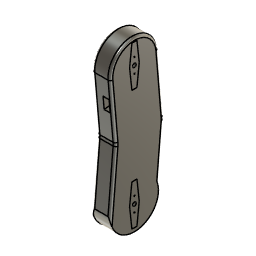
Lower-arm_segment (Autodesk Fusion 360 design; units mm, degrees)
Autodesk Fusion 360 part; units mm, degrees
note: some values were not read from the file. Chosen so that the rebuilt part matches the saved one: which face or edge a step refers to. Set by a fixed rule: which sketch regions a step uses.
sketch "Sketch1" plane through (0, 0, 0) normal (1, 0, 0) x (0, 1, 0)
  circle A0 centre (0, 0) radius 20
  circle A1 centre (0, 0) radius 1.5
  line L0 (0, 0) -> (4, 0)
  line L1 (0, 0) -> (-4, 0)
  line L2 (0, 0) -> (0, 17)
  line L3 (0, 17) -> (-2.1, 17)
  line L4 (0, 17) -> (2.1, 17)
  line L5 (-2.1, 17) -> (-4, 0)
  line L6 (2.1, 17) -> (4, 0)
  line L7 (-2.1, -17) -> (-4, 0)
  line L8 (0, -17) -> (2.1, -17)
  line L9 (0, -17) -> (-2.1, -17)
  line L10 (2.1, -17) -> (4, 0)
  line L11 (0, 0) -> (0, 6)
  line L12 (0, 0) -> (0, -6)
  circle A2 centre (0, 6) radius 0.5
  circle A3 centre (0, -6) radius 0.5
  line L13 (0, 0) -> (0, 8.5)
  line L14 (0, 0) -> (0, 100)
  line L15 (0, 0) -> (0, 50)
  line L16 (-6.3086, 50) -> (9.6914, 50)
  line L17 (2.1, 83) -> (4, 100)
  line L18 (0, 83) -> (2.1, 83)
  line L19 (0, 83) -> (-2.1, 83)
  line L20 (-2.1, 83) -> (-4, 100)
  line L21 (2.1, 117) -> (4, 100)
  line L22 (-2.1, 117) -> (-4, 100)
  line L23 (0, 117) -> (-2.1, 117)
  line L24 (0, 117) -> (2.1, 117)
  circle A4 centre (0, 100) radius 1.5
  circle A5 centre (0, 106) radius 0.5
  circle A6 centre (0, 94) radius 0.5
  circle A7 centre (0, 100) radius 20
  line L25 (-20, 0) -> (-15.741, 48.6808)
  line L26 (-20, 0) -> (10, 0) construction
  line L27 (20, 0) -> (24.261, 48.7037)
  line L28 (20, 0) -> (55, 0) construction
  line L29 (-19.9211, 98.2256) -> (-15.7431, 51.319)
  line L30 (19.9264, 101.7139) -> (24.2629, 51.2965)
  arc A8 (-15.741, 48.6808) -> (-15.7431, 51.319) centre (-30.6839, 49.9882) ccw
  arc A9 (24.261, 48.7037) -> (24.2629, 51.2965) centre (9.3181, 50.011) ccw
  line L31 (20, 0) -> (-20, 0)
  point P0 (-15.6256, 50)
  point P1 (24.3744, 50)
  dimension "d1" = 40
  dimension "d5" = 3
  dimension "d6" = 4
  dimension "d7" = 4
  dimension "d8" = 17
  dimension "d9" = 2.1
  dimension "d10" = 2.1
  dimension "d11" = 6
  dimension "d12" = 6
  dimension "d13" = 1
  dimension "d14" = 1
  dimension "d15" = 100
  dimension "d16" = 50
  dimension "d17" = 85
  dimension "d19" = 85
  dimension "d21" = 15
  dimension "d22" = 15
  constraint coincident A0.centre A1.centre
  constraint horizontal L0
  constraint parallel L0 L1
  constraint vertical L2
  constraint perpendicular L2 L3
  constraint perpendicular L2 L4
  constraint symmetric L6.end L0 L10.end
  constraint symmetric L0 L1.end L5.end
  constraint symmetric L0 L2.end L8.start
  constraint symmetric L0 L3.end L7.start
  constraint symmetric L0 L4.end L8.end
  constraint perpendicular L1 L11
  constraint perpendicular L1 L12
  constraint coincident L11.end A2.centre
  constraint coincident L12.end A3.centre
  constraint midpoint L2 L13.end
  constraint parallel L13 L14
  constraint parallel L14 L15
  constraint perpendicular L15 L16
  constraint coincident L15.end L16
  constraint symmetric A0 L16 A7
  constraint symmetric A1 L16 A4
  constraint symmetric L0.end L16 L17.end
  constraint symmetric L1.end L16 L20.end
  constraint symmetric L2.end L16 L18.start
  constraint symmetric L3.end L16 L19.end
  constraint symmetric L4.end L16 L17.start
  constraint symmetric L7.start L16 L22.start
  constraint symmetric L8.start L16 L23.start
  constraint symmetric L8.end L16 L21.start
  constraint symmetric A2 L16 A6
  constraint symmetric A3 L16 A5
  constraint horizontal L26
  constraint coincident A0 L25.start
  constraint horizontal L28
  constraint coincident A0 L27.start
  constraint coincident A7 L29.start
  constraint coincident A7 L30.start
  constraint coincident P0 L29
  constraint coincident P0 L25
  constraint tangent L29 A8
  constraint tangent L25 A8
  constraint coincident P1 L30
  constraint coincident P1 L27
  constraint tangent L30 A9
  constraint tangent L27 A9
  constraint tangent A7 L29
  constraint tangent A7 L30
  constraint coincident L16 P1
  constraint coincident L16 P0
  constraint horizontal L31
  constraint coincident A0.centre L31
  constraint coincident L27 L28.start
  constraint coincident L25 L26.start
  measures "d1" diameter of A0
  measures "d5" diameter of A1
  measures "d6" distance of A0.centre L0.end
  measures "d7" distance of A0.centre L1.end
  measures "d8" distance of A0.centre L2.end
  measures "d9" distance of L2.end L3.end
  measures "d10" distance of L2.end L4.end
  measures "d11" distance of A0.centre L11.end
  measures "d12" distance of A0.centre L12.end
  measures "d13" diameter of A2
  measures "d14" diameter of A3
  measures "d15" distance of A0.centre L14.end
  measures "d16" distance of A0.centre L15.end
  measures "d17" angle of L25 L26
  measures "d19" angle of L27 L28
  measures "d21" radius of A8
  measures "d22" radius of A9
extrude "Extrude2" add sketch "Sketch1" against normal blind 11.8 contours A1 L1 L2 L3 L5 L11 A2 L13 L14 L15 L31 | A1 L0 L1 L7 L8 L9 L10 L31 | A1 L0 L2 L4 L6 L11 A2 L13 L14 L15 L31 | L17 L18 L19 L20 L21 L22 L23 L24 makes body 1 at (-7.8667, -2.7333, 88.6667) makes body 2 at (-3.9333, -2.7333, 11.3333)
extrude "Extrude10" add sketch "Sketch1" against normal blind 15 separate body contours A0 L7 L8 L9 L10 L31 | A0 L3 L5 L14 L15 L25 L31 | A0 L4 L6 L14 L15 L31 | A0 L14 L15 A7 L27 L30 A9 | A0 L14 L15 A7 L25 L29 A8 | A7 makes body 3
sketch "Sketch12" plane through (0, -11.084, -0.9873) normal (0, -0.996057, -0.088721) x (1, 0, 0)
  line L0 (0, 52.5133) -> (0, 99.6057)
  line L1 (0, 99.6057) -> (-15, 99.6057)
  line L2 (-15, 99.6057) -> (-15, 52.5133)
  line L3 (-15, 52.5133) -> (0, 52.5133)
  line L4 (-15, 84.6057) -> (0, 84.6057)
  line L5 (-15, 84.6057) -> (-7.5, 84.6057)
  line L6 (-7.5, 84.6057) -> (-2.5, 84.6057)
  line L7 (-7.5, 84.6057) -> (-7.5, 74.6057)
  line L8 (-2.5, 84.6057) -> (-2.5, 74.6057)
  line L9 (-7.5, 74.6057) -> (-2.5, 74.6057)
  dimension "d72" = 15
  dimension "d73" = 7.5
  dimension "d74" = 5
  dimension "d75" = 10
  constraint coincident L2 L4.start
  constraint coincident L0 L4.end
  constraint perpendicular L0 L4
  constraint horizontal L5
  constraint perpendicular L0 L6
  constraint perpendicular L6 L7
  constraint perpendicular L6 L8
  constraint perpendicular L8 L9
  measures "d72" distance of L1 L4
  measures "d73" distance of L4.start L5.end
  measures "d74" distance of L5.end L6.end
  measures "d75" distance of L5.end L7.end
extrude "Extrude14" cut sketch "Sketch12" against normal blind 10 contours L4 L6 L7 L8 L9 bodies 3
sketch "Sketch13" plane through (0, -6.6191, 74.3114) normal (0, -0.088721, 0.996057) x (1, 0, 0)
  line L0 (-7.5, -11.1279) -> (-2.5, -11.1279)
  line L1 (-2.5, -11.1279) -> (-2.5, -1.1279)
  line L2 (-2.5, -1.1279) -> (-7.5, -1.1279)
  line L3 (-7.5, -1.1279) -> (-7.5, -11.1279)
  line L4 (-7.5, -6.1279) -> (-2.5, -6.1279)
  constraint midpoint L3 L4.start
  constraint midpoint L1 L4.end
extrude "Extrude15" cut sketch "Sketch13" against normal blind 50 contours L1 L2 L3 L4 bodies 3
sketch "Sketch14" plane through (-15, 0, 0) normal (-1, 0, 0) x (0, -1, 0)
  line L0 (2.1, 117) -> (4, 100)
  line L1 (4, 100) -> (2.1, 83)
  line L2 (2.1, 83) -> (-2.1, 83)
  line L3 (-2.1, 83) -> (-4, 100)
  line L4 (-4, 100) -> (-2.1, 117)
  line L5 (-2.1, 117) -> (2.1, 117)
  line L6 (2.1, -17) -> (-2.1, -17)
  line L7 (-2.1, -17) -> (-4, 0)
  line L8 (-4, 0) -> (-2.1, 17)
  line L9 (-2.1, 17) -> (2.1, 17)
  line L10 (2.1, 17) -> (4, 0)
  line L11 (4, 0) -> (2.1, -17)
  arc A0 (-20, 0) -> (20, 0) centre (0, 0) ccw
  line L12 (20, 0) -> (15.741, 48.6808)
  arc A1 (15.7431, 51.319) -> (15.741, 48.6808) centre (30.6839, 49.9882) ccw
  line L13 (15.7431, 51.319) -> (19.9211, 98.2256)
  arc A2 (19.9211, 98.2256) -> (-19.9264, 101.7139) centre (0, 100) ccw
  line L14 (-19.9264, 101.7139) -> (-24.2629, 51.2965)
  arc A3 (-24.2629, 51.2965) -> (-24.261, 48.7037) centre (-9.3181, 50.011) ccw
  line L15 (-24.261, 48.7037) -> (-20, 0)
  line L16 (3.7199, 34.6553) -> (3.7199, 24.6553)
  line L17 (3.7199, 24.6553) -> (8.7199, 24.6553)
  line L18 (8.7199, 24.6553) -> (8.7199, 34.6553)
  line L19 (8.7199, 34.6553) -> (3.7199, 34.6553)
  dimension "d83" = 5
  dimension "d84" = 10
  dimension "d85" = 10
  dimension "d86" = 5
  constraint perpendicular L16 L17
  constraint vertical L18
  constraint horizontal L19
  constraint perpendicular L16 L19
  measures "d83" distance of L18.end L16.start
  measures "d84" distance of L17.end L18.end
  measures "d85" vertical distance of L16.start L16.end
  measures "d86" horizontal distance of L16.end L17.end
extrude "Extrude16" cut sketch "Sketch14" against normal blind 10 contours L16 L17 L18 L19 bodies 3
fillet "Fillet4" radius 2 14 edges at (0, -17.8705, 24.3404) (-15, -17.8705, 24.3404) (0, -15.6839, 50) (-15, -15.6839, 50) (0, 22.1305, 24.3518) (0, 24.3181, 50) (0, 22.0947, 76.5052) (0, -1.7442, 119.9238) (0, -17.8321, 74.7723) (-15, -17.8321, 74.7723) (-15, 22.1305, 24.3518) (-15, -1.7442, 119.9238) (-15, 24.3181, 50) (-15, 22.0947, 76.5052) on bodies 3
equation "d25 = -15 mm + 3.2 mm"
